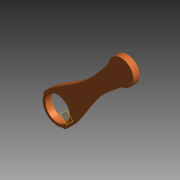
# Autodesk Inventor part: body_11
Saved by Autodesk Inventor 2013 (Build 170138000, 138)
## iProperties
Created: 2013-02-19
Part Number: body_11
Material: Wood (Cherry)
Document SubType Name: Modeling
Designer: Nano
Density: 0.5 g/cm^3
Mass: 10362.4 g
Surface Area: 8680.99 cm^2
Volume: 20724.8 cm^3
Author: Nano
Autodesk Inventor part; units mm, degrees
ref_plane "YZ Plane" through (0, 0, 0) normal (1, 0, 0) x (0, 1, 0)
ref_plane "XZ Plane" through (0, 0, 0) normal (0, 1, 0) x (-1, 0, 0)
ref_plane "XY Plane" through (0, 0, 0) normal (0, 0, 1) x (1, 0, 0)
ref_plane "Work Plane1" through (-35.1299, -83.394, 0) normal (0, 0, 1) x (0.7062905, -0.7079221, 0)
sketch "Sketch1" plane through (-35.1299, -83.394, 0) normal (0, 0, 1) x (0.7062905, -0.7079221, 0)
  circle A0 centre (-118.0078, -0.3279) radius 6.35 projected
  circle A1 centre (-118.5314, 0) radius 149.2286
  arc A2 (48.5793, -75.4462) -> (-285.6421, -75.4462) centre (-118.5314, 0) ccw
  line L0 (-118.5314, 0) -> (-118.5314, 1222.8979) construction
  arc A3 (-244.8846, 1019.4057) -> (7.8218, 1019.4057) centre (-118.5314, 1104.615) ccw
  spline S0 degree 4 poles (7.8218, 1019.4057) (-6.9781, 997.4595) (-39.0532, 578.2178) (-64.4023, 532.3679) (128.916, -51.9504) (48.5793, -75.4462) knots 0 0 0 0 0 0.373535 1 1 1 1 1
  line L1 (25.7608, 1046.0066) -> (-10.1171, 992.8047) construction
  arc A4 (19.6566, 1024.5678) -> (7.4714, 1006.4989) centre (17.8001, 1012.6766) ccw construction
  spline S1 degree 4 poles (-244.8846, 1019.4057) (-230.0846, 997.4595) (-198.0095, 578.2178) (-172.6604, 532.3679) (-365.9787, -51.9504) (-285.6421, -75.4462) knots 0 0 0 0 0 0.373535 1 1 1 1 1
  line L2 (-262.8235, 1046.0066) -> (-226.9456, 992.8047) construction
  arc A5 (-244.5341, 1006.4989) -> (-256.7193, 1024.5678) centre (-254.8628, 1012.6766) ccw construction
  arc A6 (-285.6421, -75.4462) -> (48.5793, -75.4462) centre (-118.5314, 0) ccw
  arc A7 (7.8218, 1019.4057) -> (-244.8846, 1019.4057) centre (-118.5314, 1104.615) ccw
  point P0 (-34.2245, 83.7696)
  point P1 (-21.2914, 810.23)
  point P2 (-21.2914, 520.0523)
  point P3 (59.9573, 110.7433)
  point P4 (-215.7713, 810.23)
  point P5 (-215.7713, 520.0523)
  point P6 (-297.02, 110.7433)
  dimension "d0" = 304.8
  constraints: 10 point on circle, 10 symmetric about line, 7 centre point, 6 end point, 3 midpoint, 2 tangent, 19 other
  measures "d0" diameter of A3
extrude "Extrusion1" add sketch "Sketch1" against normal blind 76.2 contours A6 A2 | A2 S1 A3 S0 | A3 A7
body "Solid1"
